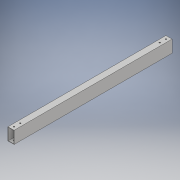
# Autodesk Inventor part: 1x2 piston attachment
Saved by Autodesk Inventor 2018 (Build 220112000, 112)
## iProperties
Created: 2019-01-29
Part Number: 1x2 piston attachment
Material: Generic
Document SubType Name: Modeling
Designer: maste
Density: 1 g/cm^3
Appearance: Default
Author: maste
Autodesk Inventor part; units mm, degrees
ref_plane "YZ Plane" through (0, 0, 0) normal (1, 0, 0) x (0, 1, 0)
ref_plane "XZ Plane" through (0, 0, 0) normal (0, 1, 0) x (-1, 0, 0)
ref_plane "XY Plane" through (0, 0, 0) normal (0, 0, 1) x (1, 0, 0)
sketch "Sketch1" plane through (0, 0, 0) normal (0, 0, 1) x (1, 0, 0)
  line L0 (0, 0) -> (25.4, 0)
  line L1 (25.4, 0) -> (25.4, 50.8)
  line L2 (25.4, 50.8) -> (0, 50.8)
  line L3 (0, 50.8) -> (0, 0)
  line L4 (1.5875, 49.2125) -> (23.8125, 49.2125)
  line L5 (23.8125, 49.2125) -> (23.8125, 1.5875)
  line L6 (23.8125, 1.5875) -> (1.5875, 1.5875)
  line L7 (1.5875, 1.5875) -> (1.5875, 49.2125)
  dimension "d0" = 25.4
  dimension "d1" = 50.8
  dimension "d2" = 1.5875
  constraints: 16 end point, 4 parallel, 2 perpendicular, 1 horizontal, 3 other
  measures "d0" distance of L2.end L1.end
  measures "d1" distance of L1.end L0.end
  measures "d2" distance between parallel lines of L2 L4
extrude "Extrusion1" add sketch "Sketch1" along normal blind 653.34
sketch "Sketch2" plane through (0, 50.8, 0) normal (0, 1, 0) x (1, 0, 0)
  line L0 (25.4, 0) -> (0, 0) construction
  line L1 (12.7, 0) -> (12.7, -12.7) construction
  line L2 (12.7, -12.7) -> (12.7, -38.1) construction
  line L3 (0, -653.34) -> (25.4, -653.34) construction
  line L4 (12.7, -653.34) -> (12.7, -640.64) construction
  line L5 (12.7, -640.64) -> (12.7, -615.24) construction
  circle A0 centre (12.7, -640.64) radius 2.5797
  circle A1 centre (12.7, -615.24) radius 2.5797
  circle A2 centre (12.7, -38.1) radius 2.5797
  circle A3 centre (12.7, -12.7) radius 2.5797
  dimension "d5" = 12.7
  dimension "d6" = 25.4
  dimension "d7" = 12.7
  dimension "d8" = 25.4
  dimension "d9" = 5.1594
  constraints: 8 end point, 4 centre point, 4 coincident, 2 midpoint, 2 point on line, 2 vertical
  measures "d5" distance of L1.start L1.end
  measures "d6" distance of L1.end L2.end
  measures "d7" distance of L4.start L4.end
  measures "d8" distance of L4.end L5.end
  measures "d9" diameter of A0
extrude "Extrusion2" cut sketch "Sketch2" against normal blind 653.34
body "Solid1"
